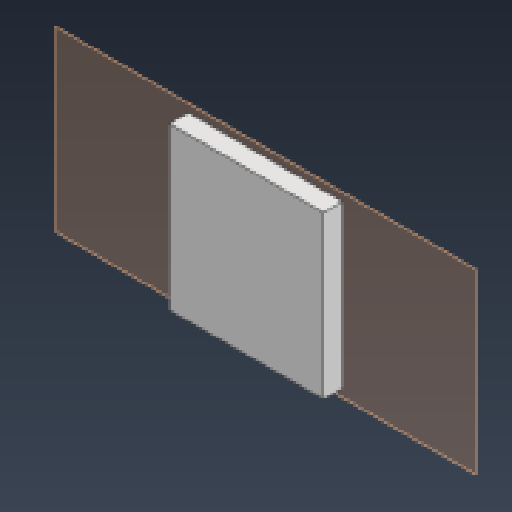
# Autodesk Inventor part: piny_led_bateryjki
Saved by Autodesk Inventor 2023 (Build 270158000, 158)
## iProperties
Created: 2025-12-26
Part Number: piny_led_bateryjki
Material: Generic
Document SubType Name: Modeling
Designer: szymo
Density: 1 g/cm^3
Appearance: Default
Author: szymo
Autodesk Inventor part; units mm, degrees
ref_plane "YZ Plane" through (0, 0, 0) normal (1, 0, 0) x (0, 1, 0)
ref_plane "XZ Plane" through (0, 0, 0) normal (0, 1, 0) x (-1, 0, 0)
ref_plane "XY Plane" through (0, 0, 0) normal (0, 0, 1) x (1, 0, 0)
ref_plane "Work Plane1" through (0, 0, 0) normal (0, 0, 1) x (1, 0, 0)
sketch "Sketch1" plane through (0, 0, 0) normal (0, 0, 1) x (1, 0, 0)
  line L0 (27, -1) -> (1, -1) projected
  line L1 (1, -1) -> (1, -12) projected
  line L2 (1, -12) -> (27, -12) projected
  line L3 (27, -12) -> (27, -1) projected
  line L4 (19.25, -12) -> (8.75, -12)
  line L5 (8.75, -12) -> (8.75, -1)
  line L6 (8.75, -1) -> (19.25, -1)
  line L7 (19.25, -1) -> (19.25, -12)
  point P0 (0, 0)
  point P1 (8.75, -1)
  dimension "d0" = 10.5
  dimension "d1" = 11
  dimension "d2" = 7.75
  constraints: 8 end point, 2 parallel, 1 horizontal, 1 perpendicular, 1 point on line
  measures "d0" distance of L5.end L6.end
  measures "d1" distance of L4.end L5.end
  measures "d2" distance between parallel lines of L7 L3
extrude "Extrusion1" add sketch "Sketch1" along normal blind 1.3 contours L7 L2 L5 L0
body "Solid1"
